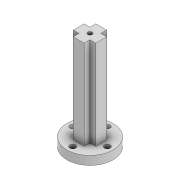
# Autodesk Inventor part: XC330_motor_adaptor
Saved by Autodesk Inventor 2022 (Build 260153000, 153)
## iProperties
Created: 2022-07-07
Part Number: XC330_motor_adaptor
Material: Generic
Document SubType Name: Modeling
Designer: dell
Density: 1 g/cm^3
Appearance: Default
Author: dell
Autodesk Inventor part; units mm, degrees
ref_plane "YZ Plane" through (0, 0, 0) normal (1, 0, 0) x (0, 1, 0)
ref_plane "XZ Plane" through (0, 0, 0) normal (0, 1, 0) x (-1, 0, 0)
ref_plane "XY Plane" through (0, 0, 0) normal (0, 0, 1) x (1, 0, 0)
sketch "Sketch1" plane through (0, 0, 0) normal (0, 1, 0) x (-1, 0, 0)
  circle A0 centre (0, 0) radius 8
  dimension "d0" = 16
  constraints: 1 centre point, 1 coincident
  measures "d0" diameter of A0
extrude "Extrusion1" add sketch "Sketch1" along normal blind 3
sketch "Sketch2" plane through (0, 3, 0) normal (0, 1, 0) x (1, 0, 0)
  circle A0 centre (-6, 0) radius 1
  point P0 (0, 0)
  dimension "d3" = 2
  dimension "d4" = 6
  constraints: 1 centre point
  measures "d3" diameter of A0
  measures "d4" distance of point (0, 0) A0.centre
extrude "Extrusion2" cut sketch "Sketch2" against normal blind 3
pattern_circular "Circular Pattern1" count 4 over 360 about axis through (0, -10, 0) along (0, 1, 0) of "Extrusion2"
sketch "Sketch3" plane through (0, 3, 0) normal (0, 1, 0) x (1, 0, 0)
  line L0 (3.9, 3.9) -> (-3.9, 3.9)
  line L1 (-3.9, 3.9) -> (-3.9, -3.9)
  line L2 (-3.9, -3.9) -> (3.9, -3.9)
  line L3 (3.9, -3.9) -> (3.9, 3.9)
  line L4 (3.9, 3.9) -> (-3.9, -3.9) construction
  line L5 (-3.9, 3.9) -> (3.9, -3.9) construction
  line L6 (-3.9, -3.9) -> (-1.9, -3.9)
  line L7 (-1.9, -3.9) -> (-1.9, -1.9)
  line L8 (-1.9, -1.9) -> (-3.9, -1.9)
  line L9 (-3.9, -1.9) -> (-3.9, -3.9)
  line L10 (-3.9, 3.9) -> (-1.9, 3.9)
  line L11 (-1.9, 3.9) -> (-1.9, 1.9)
  line L12 (-1.9, 1.9) -> (-3.9, 1.9)
  line L13 (-3.9, 1.9) -> (-3.9, 3.9)
  line L14 (3.9, -3.9) -> (1.9, -3.9)
  line L15 (1.9, -3.9) -> (1.9, -1.9)
  line L16 (1.9, -1.9) -> (3.9, -1.9)
  line L17 (3.9, -1.9) -> (3.9, -3.9)
  line L18 (3.9, 3.9) -> (1.9, 3.9)
  line L19 (1.9, 3.9) -> (1.9, 1.9)
  line L20 (1.9, 1.9) -> (3.9, 1.9)
  line L21 (3.9, 1.9) -> (3.9, 3.9)
  point P0 (0, 0)
  point P1 (3.9, 1.9)
  point P2 (1.9, 3.9)
  point P3 (-1.9, 3.9)
  point P4 (-1.9, -3.9)
  point P5 (1.9, -3.9)
  dimension "d10" = 7.8
  dimension "d11" = 7.8
  dimension "d14" = 2
  dimension "d15" = 2
  constraints: 44 end point, 10 parallel, 6 point on line, 5 horizontal, 5 perpendicular, 2 midpoint
  measures "d10" distance of L2.end L1.end
  measures "d11" distance of L1.end L0.end
  measures "d14" distance between parallel lines of L2 L16
  measures "d15" distance between parallel lines of L3 L19
extrude "Extrusion3" add sketch "Sketch3" along normal blind 31 contours L19 L20 L3 L16 L15 L2 L7 L8 L1 L12 L11 L0
sketch "Sketch4" plane through (0, 34, 0) normal (0, 1, 0) x (1, 0, 0)
  circle A0 centre (0, 0) radius 0.75
  dimension "d16" = 1.5
  constraints: 1 centre point, 1 coincident
  measures "d16" diameter of A0
extrude "Extrusion4" cut sketch "Sketch4" against normal blind 8
body "Solid1"
